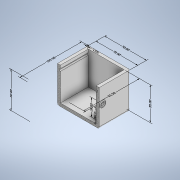
# Autodesk Inventor part: Part_A1
Saved by Autodesk Inventor 2022.6 (Build 266554010, 554A)
## iProperties
Created: 2025-05-14
Part Number: Part_A1
Material: Generic
Document SubType Name: Modeling
Designer: khinm
Density: 1 g/cm^3
Appearance: Default
Author: khinm
Autodesk Inventor part; units mm, degrees
ref_plane "YZ Plane" through (0, 0, 0) normal (1, 0, 0) x (0, 1, 0)
ref_plane "XZ Plane" through (0, 0, 0) normal (0, 1, 0) x (-1, 0, 0)
sketch "Sketch1" plane through (0, 0, 0) normal (0, 0, 1) x (1, 0, 0)
  line L0 (-35, 30) -> (35, 30)
  line L1 (35, 30) -> (35, -30)
  line L2 (35, -30) -> (-35, -30)
  line L3 (-35, -30) -> (-35, 30)
  point P0 (0, 0)
  point P1 (0, 30)
  point P2 (-35, 0)
  dimension "d0" = 70
  dimension "d1" = 60
  constraints: 8 end point, 2 midpoint, 2 parallel, 1 horizontal, 1 horizontal alignment, 1 perpendicular, 1 vertical alignment
  measures "d0" distance of L0.start L0.end
  measures "d1" distance of L0.end L1.end
extrude "Extrusion1" add sketch "Sketch1" along normal mid plane 103.5
sketch "Sketch2" plane through (-35, 30, 51.75) normal (0, 1, 0) x (1, 0, 0)
  line L0 (0, 103.5) -> (70, 103.5) projected
  line L1 (5, 98.5) -> (65, 98.5)
  line L2 (65, 98.5) -> (65, 5)
  line L3 (65, 5) -> (5, 5)
  line L4 (5, 5) -> (5, 98.5)
  point P0 (35, 51.75)
  point P1 (5, 51.75)
  point P2 (35, 98.5)
  point P3 (35, 103.5)
  dimension "d4" = 93.5
  dimension "d5" = 60
  constraints: 8 end point, 3 midpoint, 2 parallel, 1 horizontal, 1 horizontal alignment, 1 perpendicular, 1 vertical alignment
  measures "d4" distance between parallel lines of L3 L1
  measures "d5" distance of L2.end L3.end
extrude "Extrusion2" cut sketch "Sketch2" against normal blind 55
fillet "Fillet2" radius 3 8 edges at (35, 0, 51.75) (35, 0, -51.75) (-35, 0, 51.75) (-35, 0, -51.75) (35, -30, 0) (0, -30, 51.75) (-35, -30, 0) (0, -30, -51.75)
ref_plane "Work Plane1" through (0, 0, 0) normal (0, 0, 1) x (1, 0, 0)
sketch "Sketch3" plane through (0, 0, 0) normal (0, 0, 1) x (1, 0, 0)
  line L0 (-30, 30) -> (-30, -25) projected
  line L1 (-30, 25) -> (-32, 24)
  line L2 (-32, 24) -> (-32, 22)
  line L3 (-32, 30) -> (-32, -27) projected
  line L4 (-32, 22) -> (-30, 21)
  line L5 (-30, 21) -> (-30, 25)
  point P0 (0, 0)
  point P1 (-32, -25)
  dimension "d12" = 5
  dimension "d13" = 4
  dimension "d14" = 2
  dimension "d15" = 2
  constraints: 8 end point, 2 collinear, 2 point on line, 1 equal length
  measures "d12" distance of L1.start L0.start
  measures "d13" distance of L4.end L1.start
  measures "d14" distance of L2.end L1.end
  measures "d15" horizontal distance of L4.end L2.end
extrude "Extrusion3" cut sketch "Sketch3" along normal mid plane 93.5
mirror "Mirror1" about plane through (0, 0, 0) normal (1, 0, 0) of "Extrusion3"
sketch "Sketch8" plane through (35, -27, 48.75) normal (1, 0, 0) x (0, 0, -1)
  line L0 (97.5, 57) -> (0, 57) projected
  circle A0 centre (54.5, 30.5) radius 5.45
  line L1 (100.5, 0) -> (100.5, 57) projected
  line L2 (2, 2) -> (95.5, 2) projected
  point P0 (48.75, 27)
  dimension "d31" = 46
  dimension "d32" = 28.5
  dimension "d33" = 10.9
  constraints: 1 centre point
  measures "d31" distance from line of L1 A0.centre
  measures "d32" distance from line of L2 A0.centre
  measures "d33" diameter of A0
extrude "Extrusion7" add sketch "Sketch8" along normal blind 1
sketch "Sketch9" plane through (36, 3.5, -5.75) normal (1, 0, 0) x (0, 0, -1)
  circle A0 centre (0, 0) radius 5.45 projected
  circle A1 centre (0, 0) radius 2.45
  point P0 (-5.75, -3.5)
  dimension "d36" = 4.9
  constraints: 1 centre point, 1 coincident
  measures "d36" diameter of A1
extrude "Extrusion8" cut sketch "Sketch9" against normal up to surface (6 mm away) contours A1
chamfer "Chamfer1" distance 1 angle 45 3 edges at (36, 3.5, -3.3) (36, 3.5, -0.3) (30, 3.5, -3.3)
sketch "Sketch10" plane through (35, -27, 48.75) normal (1, 0, 0) x (0, 0, -1)
  line L0 (14.5, 26) -> (28.5, 26)
  line L1 (28.5, 26) -> (28.5, 37)
  line L2 (28.5, 37) -> (14.5, 37)
  line L3 (14.5, 37) -> (14.5, 26)
  line L4 (2, 48) -> (2, 2) projected
  line L5 (95.5, 2) -> (2, 2) projected
  point P0 (48.75, 27)
  dimension "d42" = 12.5
  dimension "d44" = 11
  dimension "d45" = 14
  dimension "d58" = 24
  constraints: 8 end point, 2 parallel, 1 horizontal, 1 perpendicular
  measures "d42" distance between parallel lines of L4 L3
  measures "d44" distance of L2.end L0.start
  measures "d45" distance of L0.start L0.end
  measures "d58" distance between parallel lines of L5 L0
extrude "Extrusion9" cut sketch "Sketch10" against normal blind 2
sketch "Sketch11" plane through (33, -27, 48.75) normal (1, 0, 0) x (0, 0, -1)
  line L0 (17.5, 34) -> (25.5, 34)
  line L1 (25.5, 34) -> (25.5, 29)
  line L2 (25.5, 29) -> (17.5, 29)
  line L3 (17.5, 29) -> (17.5, 34)
  line L4 (14.5, 37) -> (28.5, 37) projected
  line L5 (14.5, 26) -> (14.5, 37) projected
  point P0 (48.75, 27)
  point P1 (17.5, 31.5)
  point P2 (14.5, 31.5)
  point P3 (21.5, 37)
  point P4 (21.5, 34)
  dimension "d48" = 5
  dimension "d49" = 8
  constraints: 8 end point, 4 midpoint, 2 parallel, 1 horizontal, 1 horizontal alignment, 1 perpendicular, 1 vertical alignment
  measures "d48" distance of L1.end L0.end
  measures "d49" distance of L0.start L0.end
extrude "Extrusion10" cut sketch "Sketch11" against normal up to surface (3 mm away)
chamfer "Chamfer2" distance 1 angle 45 4 edges at (35, 10, 27.25) (35, 4.5, 20.25) (35, 4.5, 34.25) (35, -1, 27.25)
body "Solid1"
